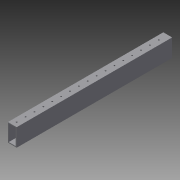
# Autodesk Inventor part: RobotBaseSide
Saved by Autodesk Inventor 2015 (Build 190159000, 159)
## iProperties
Created: 2015-10-14
Part Number: RobotBaseSide
Material: Generic
Document SubType Name: Modeling
Designer: nojessen
Density: 1 g/cm^3
Appearance: Default
Author: nojessen
Autodesk Inventor part; units mm, degrees
ref_plane "YZ Plane" through (0, 0, 0) normal (1, 0, 0) x (0, 1, 0)
ref_plane "XZ Plane" through (0, 0, 0) normal (0, 1, 0) x (-1, 0, 0)
ref_plane "XY Plane" through (0, 0, 0) normal (0, 0, 1) x (1, 0, 0)
sketch "Sketch1" plane through (0, 0, 0) normal (0, 0, 1) x (1, 0, 0)
  line L0 (0, 0) -> (25.4, 0)
  line L1 (25.4, 0) -> (25.4, 50.8)
  line L2 (25.4, 50.8) -> (0, 50.8)
  line L3 (0, 50.8) -> (0, 0)
  line L4 (22.8651, 48.2651) -> (22.8651, 2.5349)
  line L5 (22.8651, 2.5349) -> (2.5349, 2.5349)
  line L6 (2.5349, 2.5349) -> (2.5349, 48.2651)
  line L7 (2.5349, 48.2651) -> (22.8651, 48.2651)
  dimension "d0" = 25.4
  dimension "d1" = 50.8
  dimension "d2" = 2.5349
  constraints: 16 end point, 4 parallel, 2 perpendicular, 1 horizontal, 3 other
  measures "d0" distance of L2.end L1.end
  measures "d1" distance of L1.end L0.end
  measures "d2" distance between parallel lines of L1 L4
extrude "Extrusion1" add sketch "Sketch1" along normal blind 444.5
sketch "Sketch2" plane through (0, 50.8, 0) normal (0, 1, 0) x (1, 0, 0)
  line L0 (0, 0) -> (12.7, 0)
  line L1 (25.4, 0) -> (0, 0) projected
  line L2 (0, 0) -> (0, -444.5) projected
  line L3 (12.7, 0) -> (12.7, -25.4)
  circle A0 centre (12.7, -25.4) radius 1.9939
  line L4 (12.7, -25.4) -> (12.7, -50.8)
  circle A1 centre (12.7, -50.8) radius 1.9939
  line L5 (12.7, -50.8) -> (12.7, -76.2)
  circle A2 centre (12.7, -76.2) radius 1.9939
  line L6 (12.7, -25.4) -> (12.7, -50.8)
  circle A3 centre (12.7, -50.8) radius 1.9939
  line L7 (12.7, -50.8) -> (12.7, -76.2)
  circle A4 centre (12.7, -76.2) radius 1.9939
  line L8 (12.7, -76.2) -> (12.7, -101.6)
  circle A5 centre (12.7, -101.6) radius 1.9939
  line L9 (12.7, -50.8) -> (12.7, -76.2)
  circle A6 centre (12.7, -76.2) radius 1.9939
  line L10 (12.7, -76.2) -> (12.7, -101.6)
  circle A7 centre (12.7, -101.6) radius 1.9939
  line L11 (12.7, -101.6) -> (12.7, -127)
  circle A8 centre (12.7, -127) radius 1.9939
  line L12 (12.7, -76.2) -> (12.7, -101.6)
  circle A9 centre (12.7, -101.6) radius 1.9939
  line L13 (12.7, -101.6) -> (12.7, -127)
  circle A10 centre (12.7, -127) radius 1.9939
  line L14 (12.7, -127) -> (12.7, -152.4)
  circle A11 centre (12.7, -152.4) radius 1.9939
  line L15 (12.7, -101.6) -> (12.7, -127)
  circle A12 centre (12.7, -127) radius 1.9939
  line L16 (12.7, -127) -> (12.7, -152.4)
  circle A13 centre (12.7, -152.4) radius 1.9939
  line L17 (12.7, -152.4) -> (12.7, -177.8)
  circle A14 centre (12.7, -177.8) radius 1.9939
  line L18 (12.7, -127) -> (12.7, -152.4)
  circle A15 centre (12.7, -152.4) radius 1.9939
  line L19 (12.7, -152.4) -> (12.7, -177.8)
  circle A16 centre (12.7, -177.8) radius 1.9939
  line L20 (12.7, -177.8) -> (12.7, -203.2)
  circle A17 centre (12.7, -203.2) radius 1.9939
  line L21 (12.7, -152.4) -> (12.7, -177.8)
  circle A18 centre (12.7, -177.8) radius 1.9939
  line L22 (12.7, -177.8) -> (12.7, -203.2)
  circle A19 centre (12.7, -203.2) radius 1.9939
  line L23 (12.7, -203.2) -> (12.7, -228.6)
  circle A20 centre (12.7, -228.6) radius 1.9939
  line L24 (12.7, -177.8) -> (12.7, -203.2)
  circle A21 centre (12.7, -203.2) radius 1.9939
  line L25 (12.7, -203.2) -> (12.7, -228.6)
  circle A22 centre (12.7, -228.6) radius 1.9939
  line L26 (12.7, -228.6) -> (12.7, -254)
  circle A23 centre (12.7, -254) radius 1.9939
  line L27 (12.7, -203.2) -> (12.7, -228.6)
  circle A24 centre (12.7, -228.6) radius 1.9939
  line L28 (12.7, -228.6) -> (12.7, -254)
  circle A25 centre (12.7, -254) radius 1.9939
  line L29 (12.7, -254) -> (12.7, -279.4)
  circle A26 centre (12.7, -279.4) radius 1.9939
  line L30 (12.7, -228.6) -> (12.7, -254)
  circle A27 centre (12.7, -254) radius 1.9939
  line L31 (12.7, -254) -> (12.7, -279.4)
  circle A28 centre (12.7, -279.4) radius 1.9939
  line L32 (12.7, -279.4) -> (12.7, -304.8)
  circle A29 centre (12.7, -304.8) radius 1.9939
  line L33 (12.7, -254) -> (12.7, -279.4)
  circle A30 centre (12.7, -279.4) radius 1.9939
  line L34 (12.7, -279.4) -> (12.7, -304.8)
  circle A31 centre (12.7, -304.8) radius 1.9939
  line L35 (12.7, -304.8) -> (12.7, -330.2)
  circle A32 centre (12.7, -330.2) radius 1.9939
  line L36 (12.7, -279.4) -> (12.7, -304.8)
  circle A33 centre (12.7, -304.8) radius 1.9939
  line L37 (12.7, -304.8) -> (12.7, -330.2)
  circle A34 centre (12.7, -330.2) radius 1.9939
  line L38 (12.7, -330.2) -> (12.7, -355.6)
  circle A35 centre (12.7, -355.6) radius 1.9939
  line L39 (12.7, -304.8) -> (12.7, -330.2)
  circle A36 centre (12.7, -330.2) radius 1.9939
  line L40 (12.7, -330.2) -> (12.7, -355.6)
  circle A37 centre (12.7, -355.6) radius 1.9939
  line L41 (12.7, -355.6) -> (12.7, -381)
  circle A38 centre (12.7, -381) radius 1.9939
  line L42 (12.7, -330.2) -> (12.7, -355.6)
  circle A39 centre (12.7, -355.6) radius 1.9939
  line L43 (12.7, -355.6) -> (12.7, -381)
  circle A40 centre (12.7, -381) radius 1.9939
  line L44 (12.7, -381) -> (12.7, -406.4)
  circle A41 centre (12.7, -406.4) radius 1.9939
  line L45 (12.7, -355.6) -> (12.7, -381)
  circle A42 centre (12.7, -381) radius 1.9939
  line L46 (12.7, -381) -> (12.7, -406.4)
  circle A43 centre (12.7, -406.4) radius 1.9939
  line L47 (12.7, -406.4) -> (12.7, -431.8)
  circle A44 centre (12.7, -431.8) radius 1.9939
  dimension "d5" = 25.4
  dimension "d6" = 3.9878
  dimension "d7" = 25.4
  dimension "d8" = 3.9878
  dimension "d9" = 25.4
  dimension "d10" = 3.9878
  dimension "d29" = 25.4
  constraints: 92 end point, 45 centre point, 45 coincident, 4 vertical, 1 midpoint, 182 other
  measures "d5" distance of L0.end L3.end
  measures "d6" diameter of A0
  measures "d7" distance of L3.end L4.end
  measures "d8" diameter of A1
  measures "d9" distance of L4.end L5.end
  measures "d10" diameter of A2
  measures "d29" distance of L3.end L6.end
extrude "Extrusion2" cut sketch "Sketch2" against normal blind 444.5
body "Solid1"
